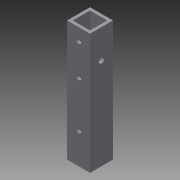
# Autodesk Inventor part: CatchSupport
Saved by Autodesk Inventor 2013 (Build 170138000, 138)
## iProperties
Created: 2014-01-24
Part Number: CatchSupport
Material: Generic
Document SubType Name: Modeling
Designer: Jarod
Density: 1 g/cm^3
Author: Jarod
Autodesk Inventor part; units mm, degrees
ref_plane "YZ Plane" through (0, 0, 0) normal (1, 0, 0) x (0, 1, 0)
ref_plane "XZ Plane" through (0, 0, 0) normal (0, 1, 0) x (-1, 0, 0)
ref_plane "XY Plane" through (0, 0, 0) normal (0, 0, 1) x (1, 0, 0)
sketch "Sketch1" plane through (0, 0, 0) normal (0, 0, 1) x (1, 0, 0)
  line L0 (0, 0) -> (25.4, 0)
  line L1 (25.4, 0) -> (25.4, 133.35)
  line L2 (25.4, 133.35) -> (0, 133.35)
  line L3 (0, 133.35) -> (0, 0)
  line L4 (25.4, 0) -> (0, 0)
  line L5 (0, 0) -> (0, 92.075)
  line L6 (0, 92.075) -> (25.4, 92.075)
  line L7 (25.4, 92.075) -> (25.4, 0)
  line L8 (12.7, 0) -> (12.7, 85.725)
  line L9 (12.7, 0) -> (98.425, 0) construction
  circle A0 centre (12.7, 85.725) radius 3.175
  line L10 (12.7, 85.725) -> (12.7, 34.925)
  circle A1 centre (12.7, 34.925) radius 3.175
  dimension "d0" = 25.4
  dimension "d1" = 133.35
  dimension "d2" = 25.4
  dimension "d3" = 92.075
  dimension "d4" = 85.725
  dimension "d5" = 90
  dimension "d6" = 6.35
  dimension "d7" = 50.8
  dimension "d8" = 6.35
  constraints: 22 end point, 5 parallel, 3 horizontal, 3 perpendicular, 2 centre point, 2 coincident, 1 midpoint, 1 point on line
  measures "d0" distance of L2.end L1.end
  measures "d1" distance of L1.end L0.end
  measures "d2" distance of L5.end L6.end
  measures "d3" distance of L4.end L5.end
  measures "d4" distance of L8.start L8.end
  measures "d5" angle of L9 L8
  measures "d6" diameter of A0
  measures "d7" distance of L10.start L10.end
  measures "d8" diameter of A1
extrude "Extrusion1" add sketch "Sketch1" along normal blind 25.4
sketch "Sketch2" plane through (0, 133.35, 0) normal (0, 1, 0) x (1, 0, 0)
  line L0 (22.225, -22.225) -> (3.175, -22.225)
  line L1 (3.175, -22.225) -> (3.175, -3.175)
  line L2 (3.175, -3.175) -> (22.225, -3.175)
  line L3 (22.225, -3.175) -> (22.225, -22.225)
  dimension "d11" = 19.05
  dimension "d12" = 19.05
  constraints: 8 end point, 2 parallel, 1 horizontal, 1 perpendicular
  measures "d11" distance of L1.end L2.end
  measures "d12" distance of L0.end L1.end
extrude "Extrusion2" cut sketch "Sketch2" against normal blind 254
sketch "Sketch3" plane through (25.4, 0, 0) normal (1, 0, 0) x (0, 0, -1)
  line L0 (0, 133.35) -> (-25.4, 133.35) projected
  line L1 (0, 0) -> (-25.4, 0) projected
  line L2 (-12.7, 133.35) -> (-12.7, 101.6)
  line L3 (-12.7, 133.35) -> (19.05, 133.35) construction
  circle A0 centre (-12.7, 101.6) radius 3.175
  dimension "d15" = 31.75
  dimension "d16" = 90
  dimension "d17" = 6.35
  constraints: 4 end point, 2 perpendicular, 1 centre point, 1 coincident, 1 horizontal, 1 midpoint
  measures "d15" distance of L2.start L2.end
  measures "d16" angle of L2 L3
  measures "d17" diameter of A0
extrude "Extrusion3" cut sketch "Sketch3" against normal blind 254
sketch "Sketch4" plane through (0, 0, 25.4) normal (0, 0, 1) x (1, 0, 0)
  line L0 (25.4, 133.35) -> (0, 133.35) projected
  line L1 (0, 133.35) -> (0, 0) projected
  line L2 (12.7, 133.35) -> (12.7, 120.65)
  line L3 (12.7, 133.35) -> (25.4, 133.35) construction
  circle A0 centre (12.7, 120.65) radius 3.175
  dimension "d20" = 12.7
  dimension "d21" = 90
  dimension "d22" = 6.35
  constraints: 4 end point, 1 centre point, 1 coincident, 1 horizontal, 1 midpoint, 1 parallel, 1 perpendicular
  measures "d20" distance of L2.start L2.end
  measures "d21" angle of L2 L3
  measures "d22" diameter of A0
extrude "Extrusion4" cut sketch "Sketch4" against normal blind 25.4
body "Solid1"
